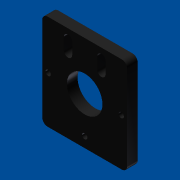
# Autodesk Inventor part: SM-S06
Saved by Autodesk Inventor 2012 SP1 (Build 160190100, 190)
## iProperties
Created: 2011-09-26
Part Number: SM-S06
Material: Polycarbonate, Smoke
Document SubType Name: Modeling
Designer: ERF
Manufacturer: Standard
Standards Organization: Custom
Density: 1.2 g/cm^3
Mass: 18.3376 g
Surface Area: 71.4211 cm^2
Volume: 15.2813 cm^3
Description: z axis mount plate
Project: Shapeoko
Vendor: ShapeOko
Stock Number: SM-S06
Subject: Structure
Author: ERF
Title: Z-Axis Mount Plate
Autodesk Inventor part; units mm, degrees
ref_plane "YZ Plane" through (0, 0, 0) normal (1, 0, 0) x (0, 1, 0)
ref_plane "XZ Plane" through (0, 0, 0) normal (0, 1, 0) x (-1, 0, 0)
ref_plane "XY Plane" through (0, 0, 0) normal (0, 0, 1) x (1, 0, 0)
sketch "Sketch1" plane through (0, 0, 0) normal (0, 0, 1) x (1, 0, 0)
  line L0 (0, 63.5) -> (50.8, 63.5)
  line L1 (50.8, 63.5) -> (50.8, 6.35)
  line L2 (50.8, 6.35) -> (0, 6.35)
  line L3 (0, 6.35) -> (0, 63.5)
  dimension "d25" = 50.8
  dimension "d26" = 57.15
  constraints: 8 end point, 2 parallel, 1 horizontal, 1 perpendicular
  measures "d25" distance of L0.start L0.end
  measures "d26" distance of L0.end L1.end
extrude "Extrusion4" add sketch "Sketch1" along normal blind 6.35
sketch "Sketch3" plane through (0, 0, 6.35) normal (0, 0, 1) x (1, 0, 0)
  line L0 (0, 63.5) -> (50.8, 63.5) projected
  line L1 (0, 6.35) -> (0, 63.5) projected
  circle A0 centre (25.4, 34.45) radius 10.625
  dimension "d29" = 21.25
  dimension "d30" = 25.4
  dimension "d31" = 29.05
  constraints: 1 centre point
  measures "d29" diameter of A0
  measures "d30" distance from line of L1 A0.centre
  measures "d31" distance from line of L0 A0.centre
extrude "Extrusion5" cut sketch "Sketch3" against normal through all
sketch "Sketch4" plane through (0, 0, 6.35) normal (0, 0, 1) x (1, 0, 0)
  line L0 (0, 63.5) -> (50.8, 63.5) projected
  line L1 (0, 6.35) -> (0, 63.5) projected
  circle A0 centre (3.49, 34.45) radius 1.6002
  circle A1 centre (47.32, 34.45) radius 1.6002
  circle A2 centre (25.4, 12.54) radius 1.6002
  dimension "d37" = 3.2004
  dimension "d38" = 3.49
  dimension "d39" = 29.05
  dimension "d40" = 3.2004
  dimension "d41" = 47.32
  dimension "d42" = 29.05
  dimension "d43" = 3.2004
  dimension "d44" = 25.4
  dimension "d45" = 50.96
  constraints: 3 centre point
  measures "d37" diameter of A0
  measures "d38" distance from line of L1 A0.centre
  measures "d39" distance from line of L0 A0.centre
  measures "d40" diameter of A1
  measures "d41" distance from line of L1 A1.centre
  measures "d42" distance from line of L0 A1.centre
  measures "d43" diameter of A2
  measures "d44" distance from line of L1 A2.centre
  measures "d45" distance from line of L0 A2.centre
extrude "Extrusion6" cut sketch "Sketch4" against normal through all
sketch "Sketch5" plane through (0, 0, 6.35) normal (0, 0, 1) x (1, 0, 0)
  line L0 (0, 63.5) -> (50.8, 63.5) projected
  line L1 (0, 6.35) -> (0, 63.5) projected
  arc A0 (12.9, 50.8) -> (17.9, 50.8) centre (15.4, 50.8) ccw
  line L2 (50.8, 6.35) -> (0, 6.35) projected
  line L3 (12.9, 50.8) -> (12.9, 57.8)
  line L4 (17.9, 50.8) -> (17.9, 57.8)
  arc A1 (17.9, 57.8) -> (12.9, 57.8) centre (15.4, 57.8) ccw
  dimension "d49" = 5
  dimension "d51" = 12.7
  dimension "d53" = 15.4
  dimension "d62" = 7
  dimension "d63" = 7
  dimension "d64" = 5
  constraints: 4 end point, 4 point on circle, 2 centre point, 2 tangent, 1 parallel, 1 perpendicular
  measures "d49" diameter of A0
  measures "d51" distance from line of L0 A0.centre
  measures "d53" distance from line of L1 A0.centre
  measures "d62" distance of L3.start L3.end
  measures "d63" distance of L4.start L4.end
  measures "d64" diameter of A1
extrude "Extrusion7" cut sketch "Sketch5" against normal through all
pattern_linear "Rectangular Pattern1" count 2 spacing 20 along (1, 0, 0) of "Extrusion7"
fillet "Fillet1" radius 3.175 4 edges at (0, 63.5, 3.175) (50.8, 63.5, 3.175) (50.8, 6.35, 3.175) (0, 6.35, 3.175)
equation "\"d40\" = d37"
equation "\"d42\" = d39"
equation "\"d43\" = d37"
equation "\"d49\" = d48"
equation "\"d63\" = d62"
equation "\"d48\" = 5"
body "Solid1"
